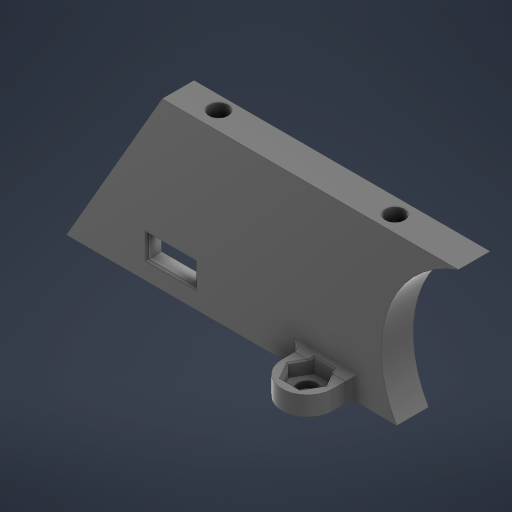
# Autodesk Inventor part: bok_lewy
Saved by Autodesk Inventor 2024 (Build 280153000, 153)
## iProperties
Created: 2024-05-25
Part Number: bok_lewy
Material: ABS Plastic
Document SubType Name: Modeling
Designer: Adam
Density: 1.06 g/cm^3
Appearance: Smooth - White
Mass: 4.70038 g
Surface Area: 30.9781 cm^2
Volume: 4.70038 cm^3
Author: Adam
Autodesk Inventor part; units mm, degrees
ref_plane "YZ Plane" through (0, 0, 0) normal (1, 0, 0) x (0, 1, 0)
ref_plane "XZ Plane" through (0, 0, 0) normal (0, 1, 0) x (-1, 0, 0)
ref_plane "XY Plane" through (0, 0, 0) normal (0, 0, 1) x (1, 0, 0)
sketch "Sketch1" plane through (0, 0, 0) normal (0, 0, 1) x (1, 0, 0)
  line L0 (15.0111, 26) -> (0, 0)
  arc A0 (61.4575, 26) -> (51.7851, 0) centre (67.3735, 9) ccw
  line L1 (61.4575, 26) -> (15.0111, 26)
  line L2 (0, 0) -> (51.7851, 0)
  dimension "d0" = 18
  dimension "d25" = 26
  constraints: 6 end point, 2 point on circle, 1 centre point, 1 coincident, 1 parallel
  measures "d0" radius of A0
  measures "d25" distance between parallel lines of L1 L2
extrude "Extrusion1" add sketch "Sketch1" along normal blind 5
sketch "Sketch4" plane through (0, 0, 0) normal (0, -1, 0) x (1, 0, 0)
  line L0 (0, 5) -> (51.7851, 5) projected
  line L1 (44.7851, 5) -> (36.7851, 5)
  line L2 (36.7851, 5) -> (36.7851, 12)
  line L3 (36.7851, 12) -> (44.7851, 12)
  line L4 (44.7851, 12) -> (44.7851, 5)
  circle A0 centre (40.7851, 8) radius 1.55
  line L5 (51.7851, 0) -> (51.7851, 5) projected
  point P0 (0, 0)
  dimension "d33" = 8
  dimension "d34" = 7
  dimension "d35" = 3.1
  dimension "d36" = 4
  dimension "d37" = 4
  dimension "d38" = 7
  constraints: 8 end point, 2 parallel, 1 centre point, 1 horizontal, 1 perpendicular, 1 point on line
  measures "d33" distance of L2.end L3.end
  measures "d34" distance of L1.end L2.end
  measures "d35" diameter of A0
  measures "d36" distance from line of L3 A0.centre
  measures "d37" distance from line of L4 A0.centre
  measures "d38" distance between parallel lines of L5 L4
extrude "Extrusion4" add sketch "Sketch4" against normal blind 3
sketch "Sketch5" plane through (0, 3, 0) normal (0, 1, 0) x (1, 0, 0)
  line L0 (42.2876, -5.3976) -> (43.7901, -8)
  line L1 (43.7901, -8) -> (42.2876, -10.6024)
  line L2 (42.2876, -10.6024) -> (39.2826, -10.6024)
  line L3 (39.2826, -10.6024) -> (37.7801, -8)
  line L4 (37.7801, -8) -> (39.2826, -5.3976)
  line L5 (39.2826, -5.3976) -> (42.2876, -5.3976)
  circle A0 centre (40.7851, -8) radius 1.55 projected
  point P0 (0, 0)
  dimension "d41" = 6.01
  constraints: 12 end point, 2 coincident, 13 other
  measures "d41" distance of L0.start L2.end
fillet "Fillet3" radius 1 3 edges at (40.7851, 3, 5) (36.7851, 1.5, 5) (44.7851, 1.5, 5)
fillet "Fillet4" radius 4 2 edges at (44.7851, 1.5, 12) (36.7851, 1.5, 12)
extrude "Extrusion5" cut sketch "Sketch5" along normal blind 3 and the other way blind 2
chamfer "Chamfer1" distance 0.2 angle 45 8 edges at (40.7851, 3.2018, 5.3976) (38.3574, 3, 7) (39.1182, 3.0518, 5.6823) (43.2127, 3, 7) (42.452, 3.0518, 5.6823) (43.0388, 3, 9.3012) (40.7851, 3, 10.6024) (38.5313, 3, 9.3012)
sketch "Sketch6" plane through (0, 0, 0) normal (0, 0, -1) x (-1, 0, 0)
  line L0 (-20.4243, 6.6958) -> (-12.4243, 6.6958)
  line L1 (-12.4243, 6.6958) -> (-12.4243, 2.6958)
  line L2 (-12.4243, 2.6958) -> (-20.4243, 2.6958)
  line L3 (-20.4243, 2.6958) -> (-20.4243, 6.6958)
  line L4 (-20.4243, 6.6958) -> (-12.4243, 2.6958) construction
  line L5 (-12.4243, 6.6958) -> (-20.4243, 2.6958) construction
  point P0 (-18.6243, 3.4939)
  point P1 (-18.6263, 5.8939)
  point P2 (-14.2243, 5.8977)
  point P3 (-14.2243, 3.4977)
  point P4 (-16.4243, 4.6958)
  dimension "d52" = 8
  dimension "d53" = 4
  constraints: 12 end point, 2 midpoint, 2 parallel, 1 horizontal, 1 perpendicular
  measures "d52" distance of L1.end L2.end
  measures "d53" distance of L0.end L1.end
extrude "Extrusion6" cut sketch "Sketch6" against normal through all
chamfer "Chamfer2" distance 2.5 distance2 4.5 4 edges at (16.4243, 6.6958, 0) (20.4243, 4.6958, 0) (16.4243, 2.6958, 0) (12.4243, 4.6958, 0) measured on face at (16.4243, 2.1958, 0) measured on face at (20.9243, 4.6958, 0) measured on face at (16.4243, 7.1958, 0) measured on face at (11.9243, 4.6958, 0)
sketch "Sketch7" plane through (15.0111, 26, 0) normal (0, 1, 0) x (1, 0, 0)
  circle A0 centre (6, -2.162) radius 1.5
  circle A1 centre (34, -2.5) radius 1.5
  line L0 (0, 0) -> (0, -5) projected
  line L1 (46.4464, 0) -> (0, 0) projected
  point P0 (-15.0111, 0)
  dimension "d59" = 3
  dimension "d60" = 3
  dimension "d61" = 6
  dimension "d62" = 28
  dimension "d63" = 2.5
  constraints: 2 centre point
  measures "d59" diameter of A0
  measures "d60" diameter of A1
  measures "d61" distance from line of L0 A0.centre
  measures "d62" horizontal distance of A0.centre A1.centre
  measures "d63" distance from line of L1 A1.centre
extrude "Extrusion7" cut sketch "Sketch7" against normal blind 2
body "Solid1"
